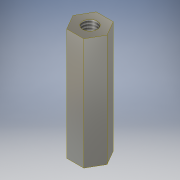
# Autodesk Inventor part: Abstandshalter_M3
Saved by Autodesk Inventor 2017 (Build 210142000, 142)
## iProperties
Part Number: Abstandshalter_M3
Material: Generisch
Document SubType Name: Modeling
Designer: ExCISS
Density: 1 g/cm^3
Appearance: Vorgabe
Author: ExCISS
Autodesk Inventor part; units mm, degrees
ref_plane "YZ Plane" through (0, 0, 0) normal (1, 0, 0) x (0, 1, 0)
ref_plane "XZ Plane" through (0, 0, 0) normal (0, 1, 0) x (-1, 0, 0)
ref_plane "XY Plane" through (0, 0, 0) normal (0, 0, 1) x (1, 0, 0)
sketch "Skizze2" plane through (0, 0, 0) normal (0, 0, 1) x (1, 0, 0)
  line L0 (-1.4434, 2.5) -> (1.4434, 2.5)
  line L1 (1.4434, 2.5) -> (2.8868, 0)
  line L2 (2.8868, 0) -> (1.4434, -2.5)
  line L3 (1.4434, -2.5) -> (-1.4434, -2.5)
  line L4 (-1.4434, -2.5) -> (-2.8868, 0)
  line L5 (-2.8868, 0) -> (-1.4434, 2.5)
  line L6 (-1.4434, 2.5) -> (1.4434, -2.5) construction
  point P0 (0, 0)
  point P1 (0, 0)
  dimension "d17" = 120
  dimension "d19" = 120
  dimension "d22" = 120
  dimension "d36" = 5
  constraints: 14 end point, 4 equal length, 2 parallel, 1 coincident, 1 horizontal, 1 midpoint
  measures "d17" angle of L0 L1
  measures "d19" angle of L1 L2
  measures "d22" angle of L3 L4
  measures "d36" distance between parallel lines of L4 L1
extrude "Extrusion1" add sketch "Skizze2" along normal mid plane 19
sketch "Skizze4" plane through (0, 0, 9.5) normal (0, 0, 1) x (1, 0, 0)
  point P0 (0, 0)
hole "Bohrung1" at (0, 0, 9.5) direction (0, 0, -1) diameter 2.459 end through all thread size "M3x0.5" class "6H" standard "ISO Metric profile"
